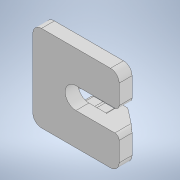
# Autodesk Inventor part: 2020 profile endcap
Saved by Autodesk Inventor 2022 (Build 260153000, 153)
## iProperties
Created: 2021-10-15
Part Number: 2020 profile endcap
Material: Generic
Document SubType Name: Modeling
Designer: tecware
Density: 1 g/cm^3
Appearance: Default
Author: tecware
## iProperties of the stored document 2020 Profile Endcap_3DPrint.ipt
Created: 2021-10-15
Part Number: 2020 Profile Endcap_3DPrint
Material: Generic
Document SubType Name: Modeling
Designer: tecware
Density: 1 g/cm^3
Appearance: Default
Author: tecware
Autodesk Inventor part; units mm, degrees
ref_plane "YZ Plane" through (0, 0, 0) normal (1, 0, 0) x (0, 1, 0)
sketch "Sketch1" plane through (0, 0, 0) normal (0, 0, 1) x (1, 0, 0)
  line L0 (-10, 10) -> (10.0183, 10)
  line L1 (10.0183, 10) -> (10.0183, -10.0055)
  line L2 (10.0183, -10.0055) -> (-10, -10.0055)
  line L3 (-10, -10.0055) -> (-10, 10)
  line L4 (-7.8, 5.3) -> (-6.987, 5.3) projected
  arc A0 (-6.2799, 5.0071) -> (-6.987, 5.3) centre (-6.987, 4.3) ccw projected
  line L5 (-6.2799, 5.0071) -> (-4.5858, 3.313) projected
  arc A1 (-4, 1.8988) -> (-4.5858, 3.313) centre (-6, 1.8988) ccw projected
  line L6 (-4, 1.8988) -> (-4, 0.3377) projected
  arc A2 (-4, 0.3377) -> (-3.9452, 0.1815) centre (-3.75, 0.3377) ccw projected
  line L7 (-3.9452, 0.1815) -> (-3.8, 0) projected
  line L8 (-3.8, 0) -> (-3.9452, -0.1815) projected
  arc A3 (-3.9452, -0.1815) -> (-4, -0.3377) centre (-3.75, -0.3377) ccw projected
  line L9 (-4, -0.3377) -> (-4, -1.8988) projected
  arc A4 (-4.5858, -3.313) -> (-4, -1.8988) centre (-6, -1.8988) ccw projected
  line L10 (-4.5858, -3.313) -> (-6.2799, -5.0071) projected
  arc A5 (-6.987, -5.3) -> (-6.2799, -5.0071) centre (-6.987, -4.3) ccw projected
  line L11 (-6.987, -5.3) -> (-7.8, -5.3) projected
  arc A6 (-8, -5.1) -> (-7.8, -5.3) centre (-7.8, -5.1) ccw projected
  line L12 (-8, -5.1) -> (-8, -3.33) projected
  arc A7 (-8, -3.33) -> (-8.25, -3.08) centre (-8.25, -3.33) ccw projected
  line L13 (-8.25, -3.08) -> (-9.75, -3.08) projected
  arc A8 (-9.75, -3.08) -> (-10, -3.33) centre (-9.75, -3.33) ccw projected
  line L14 (-10, -3.33) -> (-10, -8.5) projected
  arc A9 (-10, -8.5) -> (-8.5, -10) centre (-8.5, -8.5) ccw projected
  line L15 (-8.5, -10) -> (-3.33, -10) projected
  arc A10 (-3.33, -10) -> (-3.08, -9.75) centre (-3.33, -9.75) ccw projected
  line L16 (-3.08, -9.75) -> (-3.08, -8.25) projected
  arc A11 (-3.08, -8.25) -> (-3.33, -8) centre (-3.33, -8.25) ccw projected
  line L17 (-3.33, -8) -> (-5.1, -8) projected
  arc A12 (-5.3, -7.8) -> (-5.1, -8) centre (-5.1, -7.8) ccw projected
  line L18 (-5.3, -7.8) -> (-5.3, -6.987) projected
  arc A13 (-5.0071, -6.2799) -> (-5.3, -6.987) centre (-4.3, -6.987) ccw projected
  line L19 (-5.0071, -6.2799) -> (-3.313, -4.5858) projected
  arc A14 (-1.8988, -4) -> (-3.313, -4.5858) centre (-1.8988, -6) ccw projected
  line L20 (-1.8988, -4) -> (-0.3377, -4) projected
  arc A15 (-0.3377, -4) -> (-0.1815, -3.9452) centre (-0.3377, -3.75) ccw projected
  line L21 (-0.1815, -3.9452) -> (0, -3.8) projected
  line L22 (0, -3.8) -> (0.1815, -3.9452) projected
  arc A16 (0.1815, -3.9452) -> (0.3377, -4) centre (0.3377, -3.75) ccw projected
  line L23 (0.3377, -4) -> (1.8988, -4) projected
  arc A17 (3.313, -4.5858) -> (1.8988, -4) centre (1.8988, -6) ccw projected
  line L24 (3.313, -4.5858) -> (5.0071, -6.2799) projected
  arc A18 (5.3, -6.987) -> (5.0071, -6.2799) centre (4.3, -6.987) ccw projected
  line L25 (5.3, -6.987) -> (5.3, -7.8) projected
  arc A19 (5.1, -8) -> (5.3, -7.8) centre (5.1, -7.8) ccw projected
  line L26 (5.1, -8) -> (3.33, -8) projected
  arc A20 (3.33, -8) -> (3.08, -8.25) centre (3.33, -8.25) ccw projected
  line L27 (3.08, -8.25) -> (3.08, -9.75) projected
  arc A21 (3.08, -9.75) -> (3.33, -10) centre (3.33, -9.75) ccw projected
  line L28 (3.33, -10) -> (8.5, -10) projected
  arc A22 (8.5, -10) -> (10, -8.5) centre (8.5, -8.5) ccw projected
  line L29 (10, -8.5) -> (10, -3.33) projected
  arc A23 (10, -3.33) -> (9.75, -3.08) centre (9.75, -3.33) ccw projected
  line L30 (9.75, -3.08) -> (8.25, -3.08) projected
  arc A24 (8.25, -3.08) -> (8, -3.33) centre (8.25, -3.33) ccw projected
  line L31 (8, -3.33) -> (8, -5.1) projected
  arc A25 (7.8, -5.3) -> (8, -5.1) centre (7.8, -5.1) ccw projected
  line L32 (7.8, -5.3) -> (6.987, -5.3) projected
  arc A26 (6.2799, -5.0071) -> (6.987, -5.3) centre (6.987, -4.3) ccw projected
  line L33 (6.2799, -5.0071) -> (4.5858, -3.313) projected
  arc A27 (4, -1.8988) -> (4.5858, -3.313) centre (6, -1.8988) ccw projected
  line L34 (4, -1.8988) -> (4, -0.3377) projected
  arc A28 (4, -0.3377) -> (3.9452, -0.1815) centre (3.75, -0.3377) ccw projected
  line L35 (3.9452, -0.1815) -> (3.8, 0) projected
  line L36 (3.8, 0) -> (3.9452, 0.1815) projected
  arc A29 (3.9452, 0.1815) -> (4, 0.3377) centre (3.75, 0.3377) ccw projected
  line L37 (4, 0.3377) -> (4, 1.8988) projected
  arc A30 (4.5858, 3.313) -> (4, 1.8988) centre (6, 1.8988) ccw projected
  line L38 (4.5858, 3.313) -> (6.2799, 5.0071) projected
  arc A31 (6.987, 5.3) -> (6.2799, 5.0071) centre (6.987, 4.3) ccw projected
  line L39 (6.987, 5.3) -> (7.8, 5.3) projected
  arc A32 (8, 5.1) -> (7.8, 5.3) centre (7.8, 5.1) ccw projected
  line L40 (8, 5.1) -> (8, 3.33) projected
  arc A33 (8, 3.33) -> (8.25, 3.08) centre (8.25, 3.33) ccw projected
  line L41 (8.25, 3.08) -> (9.75, 3.08) projected
  arc A34 (9.75, 3.08) -> (10, 3.33) centre (9.75, 3.33) ccw projected
  line L42 (10, 3.33) -> (10, 8.5) projected
  arc A35 (10, 8.5) -> (8.5, 10) centre (8.5, 8.5) ccw projected
  line L43 (8.5, 10) -> (3.33, 10) projected
  arc A36 (3.33, 10) -> (3.08, 9.75) centre (3.33, 9.75) ccw projected
  line L44 (3.08, 9.75) -> (3.08, 8.25) projected
  arc A37 (3.08, 8.25) -> (3.33, 8) centre (3.33, 8.25) ccw projected
  line L45 (3.33, 8) -> (5.1, 8) projected
  arc A38 (5.3, 7.8) -> (5.1, 8) centre (5.1, 7.8) ccw projected
  line L46 (5.3, 7.8) -> (5.3, 6.987) projected
  arc A39 (5.0071, 6.2799) -> (5.3, 6.987) centre (4.3, 6.987) ccw projected
  line L47 (5.0071, 6.2799) -> (3.313, 4.5858) projected
  arc A40 (1.8988, 4) -> (3.313, 4.5858) centre (1.8988, 6) ccw projected
  line L48 (1.8988, 4) -> (0.3377, 4) projected
  arc A41 (0.3377, 4) -> (0.1815, 3.9452) centre (0.3377, 3.75) ccw projected
  line L49 (0.1815, 3.9452) -> (0, 3.8) projected
  line L50 (0, 3.8) -> (-0.1815, 3.9452) projected
  arc A42 (-0.1815, 3.9452) -> (-0.3377, 4) centre (-0.3377, 3.75) ccw projected
  line L51 (-0.3377, 4) -> (-1.8988, 4) projected
  arc A43 (-3.313, 4.5858) -> (-1.8988, 4) centre (-1.8988, 6) ccw projected
  line L52 (-3.313, 4.5858) -> (-5.0071, 6.2799) projected
  arc A44 (-5.3, 6.987) -> (-5.0071, 6.2799) centre (-4.3, 6.987) ccw projected
  line L53 (-5.3, 6.987) -> (-5.3, 7.8) projected
  arc A45 (-5.1, 8) -> (-5.3, 7.8) centre (-5.1, 7.8) ccw projected
  line L54 (-5.1, 8) -> (-3.33, 8) projected
  arc A46 (-3.33, 8) -> (-3.08, 8.25) centre (-3.33, 8.25) ccw projected
  line L55 (-3.08, 8.25) -> (-3.08, 9.75) projected
  arc A47 (-3.08, 9.75) -> (-3.33, 10) centre (-3.33, 9.75) ccw projected
  line L56 (-3.33, 10) -> (-8.5, 10) projected
  arc A48 (-8.5, 10) -> (-10, 8.5) centre (-8.5, 8.5) ccw projected
  line L57 (-10, 8.5) -> (-10, 3.33) projected
  arc A49 (-10, 3.33) -> (-9.75, 3.08) centre (-9.75, 3.33) ccw projected
  line L58 (-9.75, 3.08) -> (-8.25, 3.08) projected
  arc A50 (-8.25, 3.08) -> (-8, 3.33) centre (-8.25, 3.33) ccw projected
  line L59 (-8, 3.33) -> (-8, 5.1) projected
  arc A51 (-7.8, 5.3) -> (-8, 5.1) centre (-7.8, 5.1) ccw projected
  circle A52 centre (0, 0) radius 2.5 projected
  line L60 (0, 3.8) -> (-0.25, 4)
  line L61 (-0.25, 4) -> (-2.7272, 4)
  line L62 (-2.7272, 4) -> (-5.3, 6.5728)
  line L63 (-5.3, 6.5728) -> (-5.3, 8)
  line L64 (-5.3, 8) -> (-3.08, 8)
  line L65 (-3.08, 8) -> (-3.08, 10)
  line L66 (-3.08, 10) -> (-2.98, 10)
  line L67 (-5.3, 8) -> (-5.1, 8)
  line L68 (-2.7272, 4) -> (-2.5858, 4.1414)
  line L69 (-2.7272, 4) -> (-2.5272, 4) construction
  line L70 (-0.25, 4) -> (-0.25, 4.1)
  line L71 (0, 3.8) -> (0, 3.9)
  line L72 (0, 3.9) -> (-0.25, 4.1)
  line L73 (-5.2, 6.6142) -> (-5.2, 7.9)
  line L74 (-5.2, 7.9) -> (-2.98, 7.9)
  line L75 (-2.98, 10) -> (-2.98, 7.9)
  line L76 (-5.2, 6.6142) -> (-2.6858, 4.1)
  line L77 (-0.25, 4.1) -> (-2.6858, 4.1)
  line L78 (-10, 10) -> (0, 0)
  line L79 (-3.9, 0) -> (-4.1, 0.25)
  line L80 (-6.6142, 5.2) -> (-7.9, 5.2)
  line L81 (-7.9, 5.2) -> (-7.9, 2.98)
  line L82 (-10, 2.98) -> (-7.9, 2.98)
  line L83 (-6.6142, 5.2) -> (-4.1, 2.6858)
  line L84 (-4.1, 0.25) -> (-4.1, 2.6858)
  line L85 (0.0092, 10) -> (0.0092, -10.0055) construction
  line L86 (-10, -0.0027) -> (10.0183, -0.0027) construction
  line L87 (0, 3.9) -> (0.2683, 4.1)
  line L88 (5.2183, 6.6142) -> (5.2183, 7.9)
  line L89 (5.2183, 7.9) -> (2.9983, 7.9)
  line L90 (2.9983, 10) -> (2.9983, 7.9)
  line L91 (5.2183, 6.6142) -> (2.7041, 4.1)
  line L92 (0.2683, 4.1) -> (2.7041, 4.1)
  line L93 (4.1183, 0.25) -> (4.1183, 2.6858)
  line L94 (3.9183, 0) -> (4.1183, 0.25)
  line L95 (6.6326, 5.2) -> (4.1183, 2.6858)
  line L96 (6.6326, 5.2) -> (7.9183, 5.2)
  line L97 (7.9183, 5.2) -> (7.9183, 2.98)
  line L98 (10.0183, 2.98) -> (7.9183, 2.98)
  line L99 (0, -3.9055) -> (-0.25, -4.1055)
  line L100 (-5.2, -6.6197) -> (-5.2, -7.9055)
  line L101 (-5.2, -7.9055) -> (-2.98, -7.9055)
  line L102 (-2.98, -10.0055) -> (-2.98, -7.9055)
  line L103 (-5.2, -6.6197) -> (-2.6858, -4.1055)
  line L104 (-0.25, -4.1055) -> (-2.6858, -4.1055)
  line L105 (-4.1, -0.2555) -> (-4.1, -2.6913)
  line L106 (-3.9, 0) -> (-4.1, -0.2555)
  line L107 (-6.6142, -5.2055) -> (-4.1, -2.6913)
  line L108 (-6.6142, -5.2055) -> (-7.9, -5.2055)
  line L109 (-7.9, -5.2055) -> (-7.9, -2.9855)
  line L110 (-10, -2.9855) -> (-7.9, -2.9855)
  line L111 (0.2683, -4.1055) -> (2.7041, -4.1055)
  line L112 (0, -3.9055) -> (0.2683, -4.1055)
  line L113 (5.2183, -6.6197) -> (2.7041, -4.1055)
  line L114 (5.2183, -6.6197) -> (5.2183, -7.9055)
  line L115 (5.2183, -7.9055) -> (2.9983, -7.9055)
  line L116 (2.9983, -10.0055) -> (2.9983, -7.9055)
  line L117 (10.0183, -2.9855) -> (7.9183, -2.9855)
  line L118 (7.9183, -5.2055) -> (7.9183, -2.9855)
  line L119 (6.6326, -5.2055) -> (7.9183, -5.2055)
  line L120 (6.6326, -5.2055) -> (4.1183, -2.6913)
  line L121 (4.1183, -0.2555) -> (4.1183, -2.6913)
  line L122 (3.9183, 0) -> (4.1183, -0.2555)
  point P0 (10.0183, -10.0055)
  point P1 (10.0183, -2.9855)
  point P2 (10.0183, 2.98)
  point P3 (-10, 2.98)
  point P4 (-10, -2.9855)
  dimension "d2" = 0.1
  dimension "d7" = 45
  dimension "d8" = 0.1
  dimension "d9" = 0.1
  dimension "d24" = 0.1
  dimension "d25" = 0.1
  dimension "d26" = 0.1
  constraints: 128 end point, 45 symmetric about line, 9 point on line, 3 vertical, 2 horizontal, 1 equal length, 1 midpoint, 1 parallel, 1 perpendicular, 1 point on circle, 14 other
  measures "d2" distance of L65.end L66.end
  measures "d7" angle of L69 L68
  measures "d8" distance of L60.end L70.end
  measures "d9" distance of L49.end L71.end
  measures "d24" distance between parallel lines of L54 L74
  measures "d25" distance between parallel lines of L63 L73
  measures "d26" distance between parallel lines of L52 L76
extrude "Extrusion1" add sketch "Sketch1" against normal blind 3.5 contours L82 L81 L80 L83 A1 L84 L79 L106 L105 A4 L107 L108 L109 L110 L3 | L0 L90 L89 L88 L91 A40 L92 L87 L72 L77 A43 L76 L73 L74 L75 | L83 L84 A1 | A43 L68 L77 L76 | L102 L101 L100 L103 A14 L104 L99 L112 L111 A17 L113 L114 L115 L116 L2 | A4 L105 L107 | L1 L117 L118 L119 L120 A27 L121 L122 L94 L93 A30 L95 L96 L97 L98 | L91 L92 A40 | A43 L77 L68 | L103 L104 A14 | A30 L93 L95 | A17 L111 L113 | L120 L121 A27
extrude "Extrusion2" add sketch "Sketch1" along normal blind 3 contours L78 A48 L3 | L0 A48 L78 | L0 A47 L55 A46 L54 L64 L63 L53 L62 L52 L61 L51 A42 L50 L49 A41 L48 A40 L92 L91 L47 A39 L46 A38 L45 A37 L44 A36 A35 L42 A34 L41 A33 L40 A32 L39 A31 L38 A30 L95 L93 L37 A29 L36 L35 A28 L34 A27 L121 L120 L33 A26 L32 A25 L31 A24 L30 A23 L29 A22 L28 A21 L27 A20 L26 A19 L25 A18 L24 A17 L113 L111 L23 A16 L22 L21 A15 L20 A14 L104 L103 L19 A13 L18 A12 L17 A11 L16 A10 L15 A9 L3 A8 L13 A7 L12 A6 L11 A5 L10 A4 L107 L105 L9 A3 L8 L7 A2 L6 A1 L84 L83 L5 A0 L4 A51 L59 A50 L58 A49 A48 | L0 L65 A47 | A49 L58 A50 L59 A51 L4 A0 L5 A1 L83 L80 L81 L82 L3 | L0 L75 L74 L73 L76 A43 L52 A44 L53 A45 L54 L64 L65 L55 | L82 L81 L80 L83 A1 L84 L79 L106 L105 A4 L107 L108 L109 L110 L3 | L0 L90 L89 L88 L91 A40 L92 L87 L72 L77 A43 L76 L73 L74 L75 | L65 L64 A46 | L110 L109 L108 L107 A4 L10 A5 L11 A6 L12 A7 L13 A8 L3 | L0 A36 L44 A37 L45 A38 L46 A39 L47 A40 L91 L88 L89 L90 | A45 L63 L64 | A9 L15 A10 L16 A11 L17 A12 L18 A13 L19 A14 L103 L100 L101 L102 L2 L3 | L0 L1 L98 L97 L96 L95 A30 L38 A31 L39 A32 L40 A33 L41 A34 L42 A35 | L83 L84 A1 | L76 L77 L68 L62 A43 | A43 L68 L77 L76 | A44 L62 L63 | L102 L101 L100 L103 A14 L104 L99 L112 L111 A17 L113 L114 L115 L116 L2 | A4 L105 L107 | A1 L6 A2 L7 L8 A3 L9 A4 L105 L106 L79 L84 | L1 L117 L118 L119 L120 A27 L121 L122 L94 L93 A30 L95 L96 L97 L98 | L91 L92 A40 | A43 L77 L68 | L116 L115 L114 L113 A17 L24 A18 L25 A19 L26 A20 L27 A21 L28 A22 L29 A23 L30 A24 L31 A25 L32 A26 L33 A27 L120 L119 L118 L117 L1 L2 | A40 L48 A41 L49 L71 L87 L92 | L68 L77 A43 L61 | L77 L70 L61 L51 A43 | L72 L71 L50 L60 L70 | L61 L60 A42 | L103 L104 A14 | A30 L93 L95 | A17 L111 L113 | A14 L20 A15 L21 L22 A16 L23 A17 L111 L112 L99 L104 | L120 L121 A27 | L93 L94 L122 L121 A27 L34 A28 L35 L36 A29 L37 A30 | A52
ref_plane "Work Plane1" through (-2.98, -0.0055, -3.5) normal (0, -1, 0) x (1, 0, 0)
sketch "Sketch3" plane through (-2.98, -0.0055, -3.5) normal (0, -1, 0) x (1, 0, 0)
  line L0 (10.8983, 0) -> (12.9983, 0) projected
  line L1 (12.9983, 0) -> (8.4983, 0)
  line L2 (12.9983, 3.5) -> (10.8983, 3.5) projected
  line L3 (8.4983, 0) -> (12.9983, 3.5)
  line L4 (12.9983, 0) -> (12.9983, 3.5)
  line L5 (2.98, 3.5) -> (2.98, 0) projected
  line L6 (2.98, 0) -> (2.98, 3.5454)
  line L7 (-4.9383, 0) -> (-7.0383, 0)
  line L8 (-7.0383, 0) -> (-2.5383, 0)
  line L9 (-2.5383, 0) -> (-7.0383, 3.5)
  line L10 (-7.0383, 0) -> (-7.0383, 3.5)
  point P0 (-4.9383, 3.5)
  dimension "d15" = 4.5
  constraints: 16 end point, 5 symmetric about line, 2 vertical, 1 collinear
  measures "d15" distance of L0.end L1.end
extrude "Extrusion3" cut sketch "Sketch3" along normal through all both and the other way through all
ref_plane "Work Plane2" through (0, -10.0055, 3) normal (-1, 0, 0) x (0, 0, 1)
sketch "Sketch4" plane through (0, -10.0055, 3) normal (-1, 0, 0) x (0, 0, 1)
  line L0 (-6.5, 2.1) -> (-6.5, 0) projected
  line L1 (-6.5, 0) -> (-6.5, 4.7)
  line L2 (-3, 0) -> (0, 0) projected
  line L3 (-6.5, 4.7) -> (-3, 0)
  line L4 (-3, 0) -> (-6.5, 0)
  line L5 (-3, 10.0055) -> (-6.5, 10.0055) projected
  line L6 (-6.5, 10.0055) -> (0.7885, 10.0055)
  line L7 (-6.5, 17.911) -> (-6.5, 20.011)
  line L8 (-6.5, 20.011) -> (-6.5, 15.311)
  line L9 (-6.5, 15.311) -> (-3, 20.011)
  line L10 (-3, 20.011) -> (-6.5, 20.011)
  dimension "d19" = 4.7
  constraints: 16 end point, 4 symmetric about line, 2 collinear, 1 horizontal
  measures "d19" distance of L0.end L1.end
extrude "Extrusion4" cut sketch "Sketch4" along normal through all both and the other way through all
fillet "Fillet1" radius 0.75 28 edges at (-5.2, -7.9055, -0.7819) (-7.9, -5.2055, -0.8238) (-6.6142, -5.2055, -1.3238) (-5.2, -6.6197, -1.2607) (-2.6858, -4.1055, -1.75) (2.7041, -4.1055, -1.75) (0, -3.9055, -1.75) (-3.9, 0, -1.75) (0, 3.9, -1.75) (3.9183, 0, -1.75) (4.1183, -2.6913, -1.75) (4.1183, 2.6858, -1.75) (2.7041, 4.1, -1.75) (-2.6858, 4.1, -1.75) (-4.1, -2.6913, -1.75) (-4.1, 2.6858, -1.75) (-6.6142, 5.2, -1.3238) (5.2183, 6.6142, -1.2627) (5.2183, 7.9, -0.784) (7.9183, 5.2, -0.8167) (6.6326, 5.2, -1.3167) (6.6326, -5.2055, -1.3167) (7.9183, -5.2055, -0.8167) (5.2183, -7.9055, -0.7819) (5.2183, -6.6197, -1.2607) (-7.9, 5.2, -0.8238) (-5.2, 7.9, -0.784) (-5.2, 6.6142, -1.2627)
sketch "Sketch5" plane through (0, 0, 3) normal (0, 0, 1) x (1, 0, 0)
  line L0 (10.0183, -10.0055) -> (10.0183, 10) projected
  line L1 (2.5, 0) -> (0, 0)
  circle A0 centre (0, 0) radius 2.5
  line L2 (0, 2.5) -> (10.0183, 2.5)
  line L3 (0, -2.5) -> (10.0183, -2.5)
  point P0 (0, 0)
  point P1 (10.0183, -8.0055)
  point P2 (10.0183, 8)
  dimension "d32" = 5
  dimension "d35" = 0
  constraints: 6 end point, 2 perpendicular, 2 point on circle, 2 point on line, 2 tangent, 1 centre point, 1 coincident, 1 horizontal
  measures "d32" diameter of A0
  measures "d35" distance of point (0, 0) L1.end
extrude "Extrusion5" cut sketch "Sketch5" against normal through all
fillet "Fillet3" radius 2 4 edges at (10.0183, -10.0055, 1.5) (10.0183, 10, 1.5) (-10, 10, 1.5) (-10, -10.0055, 1.5)
fillet "Fillet4" radius 1 2 edges at (10.0183, -2.5, 1.5) (10.0183, 2.5, 1.5)
equation "\"d8\" = d26"
equation "\"d9\" = d8"
equation "\"d24\" = d25"
equation "\"d25\" = d2"
equation "\"d26\" = d24"
body "Solid1"
